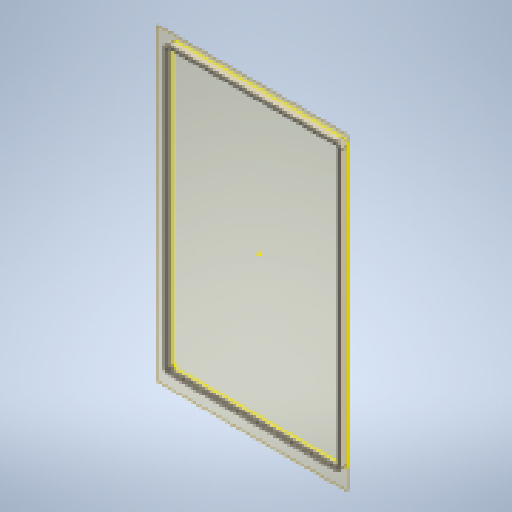
# Autodesk Inventor part: enclosure-body
Saved by Autodesk Inventor 2024 (Build 280153000, 153)
## iProperties
Created: 2024-11-18
Part Number: enclosure-body
Material: Generic
Document SubType Name: Modeling
Designer: Stefano
Density: 1 g/cm^3
Appearance: Default
Author: Stefano
Autodesk Inventor part; units mm, degrees
ref_plane "YZ Plane" through (0, 0, 0) normal (1, 0, 0) x (0, 1, 0)
ref_plane "XZ Plane" through (0, 0, 0) normal (0, 1, 0) x (-1, 0, 0)
ref_plane "XY Plane" through (0, 0, 0) normal (0, 0, 1) x (1, 0, 0)
ref_plane "Work Plane1" through (0, 0, 0) normal (0, 0, 1) x (1, 0, 0)
sketch "Sketch1" plane through (0, 0, 0) normal (0, 0, 1) x (1, 0, 0)
  arc A0 (-71.5, 119.5) -> (-73.5, 117.5) centre (-71.5, 117.5) ccw construction
  line L0 (-73.5, 117.5) -> (-73.5, -117.5) construction
  arc A1 (-73.5, -117.5) -> (-71.5, -119.5) centre (-71.5, -117.5) ccw construction
  line L1 (-71.5, -119.5) -> (71.5, -119.5) construction
  arc A2 (71.5, -119.5) -> (73.5, -117.5) centre (71.5, -117.5) ccw construction
  line L2 (73.5, -117.5) -> (73.5, 117.5) construction
  arc A3 (73.5, 117.5) -> (71.5, 119.5) centre (71.5, 117.5) ccw construction
  line L3 (71.5, 119.5) -> (-71.5, 119.5) construction
  line L4 (-67.98, 108.59) -> (67.98, 108.59) construction
  line L5 (67.98, 108.59) -> (67.98, -108.59) construction
  line L6 (67.98, -108.59) -> (-67.98, -108.59) construction
  line L7 (-67.98, -108.59) -> (-67.98, 108.59) construction
  line L8 (-73.7, -117.5) -> (-73.7, 117.5)
  arc A4 (-71.5, 119.7) -> (-73.7, 117.5) centre (-71.5, 117.5) ccw
  line L9 (-71.5, 119.7) -> (71.5, 119.7)
  arc A5 (73.7, 117.5) -> (71.5, 119.7) centre (71.5, 117.5) ccw
  line L10 (73.7, 117.5) -> (73.7, -117.5)
  arc A6 (71.5, -119.7) -> (73.7, -117.5) centre (71.5, -117.5) ccw
  line L11 (71.5, -119.7) -> (-71.5, -119.7)
  arc A7 (-73.7, -117.5) -> (-71.5, -119.7) centre (-71.5, -117.5) ccw
  line L12 (-75.7, 117.5) -> (-75.7, -117.5)
  arc A8 (-75.7, -117.5) -> (-71.5, -121.7) centre (-71.5, -117.5) ccw
  line L13 (-71.5, -121.7) -> (71.5, -121.7)
  arc A9 (71.5, -121.7) -> (75.7, -117.5) centre (71.5, -117.5) ccw
  line L14 (75.7, -117.5) -> (75.7, 117.5)
  arc A10 (75.7, 117.5) -> (71.5, 121.7) centre (71.5, 117.5) ccw
  line L15 (71.5, 121.7) -> (-71.5, 121.7)
  arc A11 (-71.5, 121.7) -> (-75.7, 117.5) centre (-71.5, 117.5) ccw
  point P0 (0, 0)
  dimension "d0" = 0.2
  dimension "d1" = 2
  constraints: 16 end point, 16 point on circle, 8 centre point, 14 other
  measures "d0" distance between parallel lines of L0 L8
  measures "d1" distance between parallel lines of L12 L8
ref_plane "Work Plane2" through (-73.5, -119.5, -1.1) normal (0, 0, -1) x (0, 1, 0)
extrude "Extrusion1" add sketch "Sketch1" against normal up to surface (1.1 mm away)
sketch "Sketch2" plane through (71.5, -121.7, -1.1) normal (0, 0, -1) x (-1, 0, 0)
  arc A0 (143, 2) -> (145.2, 4.2) centre (143, 4.2) ccw construction
  line L0 (0, 2) -> (143, 2) construction
  arc A1 (-2.2, 4.2) -> (0, 2) centre (0, 4.2) ccw construction
  line L1 (-2.2, 239.2) -> (-2.2, 4.2) construction
  arc A2 (0, 241.4) -> (-2.2, 239.2) centre (0, 239.2) ccw construction
  line L2 (143, 241.4) -> (0, 241.4) construction
  arc A3 (145.2, 239.2) -> (143, 241.4) centre (143, 239.2) ccw construction
  line L3 (145.2, 4.2) -> (145.2, 239.2) construction
  line L4 (143, 0) -> (0, 0) projected
  arc A4 (143, 0) -> (147.2, 4.2) centre (143, 4.2) ccw projected
  line L5 (147.2, 239.2) -> (147.2, 4.2) projected
  arc A5 (147.2, 239.2) -> (143, 243.4) centre (143, 239.2) ccw projected
  line L6 (0, 243.4) -> (143, 243.4) projected
  arc A6 (0, 243.4) -> (-4.2, 239.2) centre (0, 239.2) ccw projected
  line L7 (-4.2, 4.2) -> (-4.2, 239.2) projected
  arc A7 (-4.2, 4.2) -> (0, 0) centre (0, 4.2) ccw projected
  line L8 (71.5, 121.7) -> (71.5, 0) construction
  constraints: 2 end point, 1 midpoint
sketch "Sketch4" plane through (0, 0, 0) normal (1, 0, 0) x (0, 1, 0)
  line L0 (-121.7, -1.1) -> (-117.7, -1.1)
  line L1 (-117.7, -1.1) -> (-119.7, -6.1)
  line L2 (-119.7, -6.1) -> (-121.7, -6.1)
  line L3 (-121.7, -6.1) -> (-121.7, -1.1)
  point P0 (0, 0)
  point P1 (-121.7, -1.1)
  dimension "d6" = 4
  dimension "d7" = 2
  dimension "d8" = 5
  constraints: 8 end point, 1 horizontal, 1 parallel, 1 perpendicular
  measures "d6" distance of L0.start L0.end
  measures "d7" distance of L1.end L2.end
  measures "d8" distance of L2.end L0.start
sweep "Sweep1" add profiles "Sketch4" path "Sketch2" path curves L6 A6 L7 A7 L4 A4 L5 A5
sketch "Sketch5" plane through (71.5, -121.7, -6.1) normal (0, 0, -1) x (-1, 0, 0)
  arc A0 (0, 241.4) -> (-2.2, 239.2) centre (0, 239.2) ccw projected
  line L0 (143, 241.4) -> (0, 241.4) projected
  arc A1 (145.2, 239.2) -> (143, 241.4) centre (143, 239.2) ccw projected
  line L1 (145.2, 4.2) -> (145.2, 239.2) projected
  arc A2 (143, 2) -> (145.2, 4.2) centre (143, 4.2) ccw projected
  line L2 (0, 2) -> (143, 2) projected
  arc A3 (-2.2, 4.2) -> (0, 2) centre (0, 4.2) ccw projected
  line L3 (-2.2, 239.2) -> (-2.2, 4.2) projected
  line L4 (-4.2, 239.2) -> (-4.2, 4.2) projected
  arc A4 (-4.2, 4.2) -> (0, 0) centre (0, 4.2) ccw projected
  line L5 (0, 0) -> (143, 0) projected
  arc A5 (143, 0) -> (147.2, 4.2) centre (143, 4.2) ccw projected
  line L6 (147.2, 4.2) -> (147.2, 239.2) projected
  arc A6 (147.2, 239.2) -> (143, 243.4) centre (143, 239.2) ccw projected
  line L7 (143, 243.4) -> (0, 243.4) projected
  arc A7 (0, 243.4) -> (-4.2, 239.2) centre (0, 239.2) ccw projected
  point P0 (71.5, 121.7)
extrude "Extrusion2" add sketch "Sketch5" along normal blind 50.8
ref_plane "Work Plane4" through (0, 0, -9.9) normal (0, 0, -1) x (-1, 0, 0)
sketch "Sketch6" plane through (0, 0, -9.9) normal (0, 0, -1) x (-1, 0, 0)
  circle A0 centre (34, 47.5) radius 1.3 construction
  circle A1 centre (-34, 47.5) radius 1.3 construction
  circle A2 centre (-34, -47.5) radius 1.3 construction
  circle A3 centre (34, -47.5) radius 1.3 construction
  line L0 (37, 52) -> (-37, 52) construction
  line L1 (73.7, 117.5) -> (73.7, -117.5) construction
  line L2 (-73.7, -117.5) -> (-73.7, 117.5) construction
  line L3 (73.7, 77.4) -> (-73.7, 77.4)
  line L4 (-73.7, 77.4) -> (-73.7, 43.5)
  line L5 (-73.7, 43.5) -> (73.7, 43.5)
  line L6 (73.7, 43.5) -> (73.7, 77.4)
  line L7 (30, 43.5) -> (-30, 43.5)
  line L8 (-30, 43.5) -> (-30, 52)
  line L9 (-30, 52) -> (30, 52)
  line L10 (30, 52) -> (30, 43.5)
  line L11 (73.7, -43.5) -> (-73.7, -43.5)
  line L12 (-73.7, -43.5) -> (-73.7, -74.615)
  line L13 (-73.7, -74.615) -> (73.7, -74.615)
  line L14 (73.7, -74.615) -> (73.7, -43.5)
  line L15 (30, -43.5) -> (-38, -43.5)
  line L16 (-38, -43.5) -> (-38, -65.09)
  line L17 (-38, -65.09) -> (30, -65.09)
  line L18 (30, -65.09) -> (30, -43.5)
  line L19 (-38, -43.5) -> (-30, -43.5)
  line L20 (-30, -43.5) -> (-30, -51.5)
  line L21 (-30, -51.5) -> (-38, -51.5)
  line L22 (-38, -51.5) -> (-38, -43.5)
  point P0 (0, 0)
  point P1 (-30, 47.75)
  point P2 (-30, -47.5)
  dimension "d13" = 25.4
  dimension "d14" = 4
  dimension "d15" = 4
  dimension "d16" = 4
  dimension "d17" = 4
  dimension "d18" = 4
  dimension "d19" = 4
  dimension "d20" = 4
  dimension "d21" = 9.525
  dimension "d22" = 21.59
  dimension "d23" = 4
  constraints: 40 end point, 10 parallel, 7 point on line, 5 horizontal, 5 perpendicular, 2 midpoint
  measures "d13" distance between parallel lines of L3 L0
  measures "d14" distance from line of L5 A0.centre
  measures "d15" horizontal distance of point (-30, 47.75) A1.centre
  measures "d16" distance from line of L10 A0.centre
  measures "d17" distance from line of L11 A3.centre
  measures "d18" distance of point (-30, -47.5) A2.centre
  measures "d19" distance from line of L21 A2.centre
  measures "d20" distance from line of L16 A2.centre
  measures "d21" distance between parallel lines of L17 L13
  measures "d22" distance between parallel lines of L15 L17
  measures "d23" distance from line of L18 A3.centre
extrude "Extrusion3" add sketch "Sketch6" along normal blind 3 contours L6 L5 L10 L9 L8 L4 L3 | L14 L13 L12 L11 L16 L17 L18 | L20 L21 L16 L11
sketch "Sketch7" plane through (0, 0, -12.9) normal (0, 0, -1) x (-1, 0, 0)
  circle A0 centre (34, 47.5) radius 1.3 construction
  circle A1 centre (-34, 47.5) radius 1.3 construction
  circle A2 centre (-34, -47.5) radius 1.3 construction
  circle A3 centre (34, -47.5) radius 1.3 construction
  point P0 (0, 0)
hole "Hole1" at (-34, 47.5, -12.9) at (34, 47.5, -12.9) at (34, -47.5, -12.9) at (-34, -47.5, -12.9) direction (0, 0, 1) diameter 3.6068 end through all
fillet "Fillet1" radius 4 4 edges at (-30, -43.5, -11.4) (-30, 43.5, -11.4) (30, 43.5, -11.4) (30, -43.5, -11.4)
fillet "Fillet2" radius 4 14 edges at (-30, -65.09, -11.4) (38, -65.09, -11.4) (-30, 52, -11.4) (30, 52, -11.4) (30, -51.5, -11.4) (38, -51.5, -11.4) (73.7, -74.615, -11.4) (73.7, -43.5, -11.4) (73.7, 43.5, -11.4) (73.7, 77.4, -11.4) (-73.7, 77.4, -11.4) (-73.7, 43.5, -11.4) (-73.7, -43.5, -11.4) (-73.7, -74.615, -11.4)
ref_plane "Work Plane5" through (34, -47.5, -12.9) normal (0, 1, 0) x (1, 0, 0)
ref_plane "Work Plane6" through (34, 47.5, -12.9) normal (0, 1, 0) x (1, 0, 0)
sketch "Sketch8" plane through (34, 47.5, -12.9) normal (0, 1, 0) x (1, 0, 0)
  line L0 (-64, 0) -> (-64, -3) construction
  line L1 (-64, -3) -> (-66.1966, -3) construction
  line L2 (-66.1966, -3) -> (-66.1966, 0) construction
  line L3 (-66.1966, 0) -> (-64, 0) construction
  line L4 (-4, -3) -> (-4, 0) construction
  line L5 (-4, 0) -> (-1.8034, 0) construction
  line L6 (-1.8034, 0) -> (-1.8034, -3) construction
  line L7 (-1.8034, -3) -> (-4, -3) construction
  line L8 (39.7, -11.8) -> (37.7, -11.8) construction
  line L9 (37.7, -11.8) -> (39.7, -6.8) construction
  line L10 (39.7, -6.8) -> (39.7, -3) construction
  line L11 (39.7, -3) -> (1.8034, -3) construction
  line L12 (1.8034, -3) -> (1.8034, 0) construction
  line L13 (1.8034, 0) -> (39.7, 0) construction
  line L14 (39.7, 0) -> (39.7, 44) construction
  line L15 (39.7, 44) -> (41.7, 44) construction
  line L16 (41.7, 44) -> (41.7, -12.9) construction
  line L17 (41.7, -12.9) -> (39.7, -12.9) construction
  line L18 (39.7, -12.9) -> (39.7, -11.8) construction
  line L19 (-105.7, -11.8) -> (-107.7, -11.8) construction
  line L20 (-107.7, -11.8) -> (-107.7, -12.9) construction
  line L21 (-107.7, -12.9) -> (-109.7, -12.9) construction
  line L22 (-109.7, -12.9) -> (-109.7, 44) construction
  line L23 (-109.7, 44) -> (-107.7, 44) construction
  line L24 (-107.7, 44) -> (-107.7, 0) construction
  line L25 (-107.7, 0) -> (-69.8034, 0) construction
  line L26 (-69.8034, 0) -> (-69.8034, -3) construction
  line L27 (-69.8034, -3) -> (-107.7, -3) construction
  line L28 (-107.7, -3) -> (-107.7, -6.8) construction
  line L29 (-107.7, -6.8) -> (-105.7, -11.8) construction
  line L30 (39.7, 9.525) -> (11.125, 0)
  line L31 (-107.7, 9.525) -> (-79.125, 0)
  point P0 (-34, -12.9)
  dimension "d35" = 28.575
  dimension "d36" = 9.525
  dimension "d37" = 9.525
  dimension "d38" = 28.575
  constraints: 4 end point, 4 point on line
  measures "d35" distance from line of L14 L30.end
  measures "d36" distance from line of L13 L30.start
  measures "d37" distance from line of L25 L31.start
  measures "d38" distance from line of L24 L31.end
sketch "Sketch9" plane through (34, -47.5, -12.9) normal (0, 1, 0) x (1, 0, 0)
  line L0 (-4, 0) -> (-1.8034, 0) construction
  line L1 (-1.8034, 0) -> (-1.8034, -3) construction
  line L2 (-1.8034, -3) -> (-4, -3) construction
  line L3 (-4, -3) -> (-4, 0) construction
  line L4 (-64, -3) -> (-66.1966, -3) construction
  line L5 (-66.1966, -3) -> (-66.1966, 0) construction
  line L6 (-66.1966, 0) -> (-64, 0) construction
  line L7 (-64, 0) -> (-64, -3) construction
  line L8 (39.7, -11.8) -> (37.7, -11.8) construction
  line L9 (37.7, -11.8) -> (39.7, -6.8) construction
  line L10 (39.7, -6.8) -> (39.7, -3) construction
  line L11 (39.7, -3) -> (1.8034, -3) construction
  line L12 (1.8034, -3) -> (1.8034, 0) construction
  line L13 (1.8034, 0) -> (39.7, 0) construction
  line L14 (39.7, 0) -> (39.7, 44) construction
  line L15 (39.7, 44) -> (41.7, 44) construction
  line L16 (41.7, 44) -> (41.7, -12.9) construction
  line L17 (41.7, -12.9) -> (39.7, -12.9) construction
  line L18 (39.7, -12.9) -> (39.7, -11.8) construction
  line L19 (-105.7, -11.8) -> (-107.7, -11.8) construction
  line L20 (-107.7, -11.8) -> (-107.7, -12.9) construction
  line L21 (-107.7, -12.9) -> (-109.7, -12.9) construction
  line L22 (-109.7, -12.9) -> (-109.7, 44) construction
  line L23 (-109.7, 44) -> (-107.7, 44) construction
  line L24 (-107.7, 44) -> (-107.7, 0) construction
  line L25 (-107.7, 0) -> (-69.8034, 0) construction
  line L26 (-69.8034, 0) -> (-69.8034, -3) construction
  line L27 (-69.8034, -3) -> (-107.7, -3) construction
  line L28 (-107.7, -3) -> (-107.7, -6.8) construction
  line L29 (-107.7, -6.8) -> (-105.7, -11.8) construction
  line L30 (-107.7, 9.525) -> (-79.125, 0)
  line L31 (39.7, 9.525) -> (11.125, 0)
  point P0 (-34, -12.9)
  dimension "d39" = 9.525
  dimension "d40" = 28.575
  dimension "d41" = 9.525
  dimension "d42" = 28.575
  constraints: 4 end point, 4 point on line
  measures "d39" distance from line of L13 L31.start
  measures "d40" distance from line of L14 L31.end
  measures "d41" distance of L24.end L30.start
  measures "d42" distance from line of L24 L30.end
extrude "Rib1" add sketch "Sketch8" along normal mid plane 2 rib yes fills toward (25.4283, 4.7151) open curves L30
extrude "Rib2" add sketch "Sketch9" along normal mid plane 2 rib yes fills toward (25.4283, 4.7151) open curves L31
extrude "Rib3" add sketch "Sketch8" along normal mid plane 2 rib yes fills toward (-93.4283, 4.7151) open curves L31
extrude "Rib4" add sketch "Sketch9" along normal mid plane 2 rib yes fills toward (-93.4283, 4.7151) open curves L30
equation "\"d39\" = d36"
equation "\"d40\" = d35"
equation "\"d41\" = d36"
equation "\"d42\" = d35"
body "Solid1"
